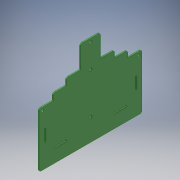
# Autodesk Inventor part: PCB
Saved by Autodesk Inventor 2017 (Build 210142000, 142)
## iProperties
Created: 2016-11-14
Part Number: PCB
Material: Generic
Document SubType Name: Modeling
Designer: Shichi
Density: 1 g/cm^3
Appearance: Smooth - Dark Forest Green
Author: Shichi
Autodesk Inventor part; units mm, degrees
ref_plane "YZ Plane" through (0, 0, 0) normal (1, 0, 0) x (0, 1, 0)
ref_plane "XZ Plane" through (0, 0, 0) normal (0, 1, 0) x (-1, 0, 0)
ref_plane "XY Plane" through (0, 0, 0) normal (0, 0, 1) x (1, 0, 0)
sketch "Sketch1" plane through (0, 0, 0) normal (1, 0, 0) x (0, 1, 0)
  line L0 (47, 25) -> (-47, 25)
  line L1 (-47, 25) -> (-47, -25)
  line L2 (-47, -25) -> (47, -25)
  line L3 (47, -25) -> (47, 25)
  circle A0 centre (44, 22) radius 1.25
  line L4 (0, 25) -> (0, -25) construction
  circle A1 centre (-44, 22) radius 1.25
  line L5 (-34, 25) -> (-34, 31)
  line L6 (-34, 31) -> (34, 31)
  line L7 (34, 31) -> (34, 25)
  line L8 (-33, -12) -> (-22, -12)
  line L9 (-22, -12) -> (-22, -13)
  line L10 (-22, -13) -> (-33, -13)
  line L11 (-33, -13) -> (-33, -12)
  line L12 (33, -12) -> (22, -12)
  line L13 (22, -12) -> (22, -13)
  line L14 (22, -13) -> (33, -13)
  line L15 (33, -13) -> (33, -12)
  line L16 (-41, 7) -> (-42, 7)
  line L17 (-42, 7) -> (-42, -4)
  line L18 (-42, -4) -> (-41, -4)
  line L19 (-41, -4) -> (-41, 7)
  line L20 (41, 7) -> (42, 7)
  line L21 (42, 7) -> (42, -4)
  line L22 (42, -4) -> (41, -4)
  line L23 (41, -4) -> (41, 7)
  circle A2 centre (0, -5) radius 1.25
  circle A3 centre (0, 54.3) radius 1.25
  line L24 (22, 31) -> (22, 37)
  line L25 (22, 37) -> (9, 37)
  line L26 (9, 37) -> (9, 57.5)
  line L27 (-9, 57.5) -> (-9, 37)
  line L28 (-9, 37) -> (-22, 37)
  line L29 (-22, 37) -> (-22, 31)
  line L30 (9, 57.5) -> (-9, 57.5)
  circle A4 centre (0, 32.7) radius 1.25
  point P0 (0, 0)
  point P1 (47, 0)
  dimension "d0" = 50
  dimension "d1" = 94
  dimension "d2" = 2.5
  dimension "d3" = 3
  dimension "d4" = 3
  dimension "d11" = 13
  dimension "d12" = 6
  dimension "d13" = 13
  dimension "d18" = 1
  dimension "d19" = 11
  dimension "d20" = 14
  dimension "d21" = 12
  dimension "d24" = 21
  dimension "d25" = 1
  dimension "d26" = 5
  dimension "d27" = 11
  dimension "d28" = 30
  dimension "d29" = 2.5
  dimension "d30" = 2.5
  dimension "d33" = 6
  dimension "d34" = 25
  dimension "d35" = 25
  dimension "d37" = 12
  dimension "d38" = 12
  dimension "d39" = 9
  dimension "d41" = 26.5
  dimension "d42" = 3.2
  dimension "d43" = 2.5
  dimension "d44" = 37.7
  constraints: 62 end point, 9 perpendicular, 9 symmetric about line, 8 point on line, 7 parallel, 5 centre point, 5 horizontal, 3 midpoint, 3 vertical alignment, 2 horizontal alignment, 1 other
  measures "d0" distance of L2.end L0.start
  measures "d1" distance of L1.end L2.end
  measures "d2" diameter of A0
  measures "d3" distance from line of A0.centre L3
  measures "d4" distance from line of L0 A0.centre
  measures "d11" distance from line of L0.end L5
  measures "d12" distance of L5.start L5.end
  measures "d13" distance from line of L7 L0.start
  measures "d18" distance between parallel lines of L10 L8
  measures "d19" distance between parallel lines of L9 L11
  measures "d20" distance from line of L1 L8.start
  measures "d21" distance between parallel lines of L2 L10
  measures "d24" distance between parallel lines of L18 L2
  measures "d25" distance between parallel lines of L19 L17
  measures "d26" distance between parallel lines of L1 L17
  measures "d27" distance of L18.end L16.start
  measures "d28" distance from line of L0 A2.centre
  measures "d29" diameter of A2
  measures "d30" diameter of A3
  measures "d33" distance of L24.start L24.end
  measures "d34" distance between parallel lines of L7 L26
  measures "d35" distance between parallel lines of L5 L27
  measures "d37" distance between parallel lines of L7 L24
  measures "d38" distance between parallel lines of L5 L29
  measures "d39" distance from line of L27 A3.centre
  measures "d41" distance between parallel lines of L6 L30
  measures "d42" distance from line of L30 A3.centre
  measures "d43" diameter of A4
  measures "d44" distance of A2.centre A4.centre
extrude "Extrusion1" add sketch "Sketch1" along normal blind 1 contours L3 L2 L1 L0 | L0 L5 L6 L7 | L6 L29 L28 L27 L30 L26 L25 L24 | L8 L9 L10 L11 | L15 L14 L13 L12 | L19 L18 L17 L16 | L20 L21 L22 L23 | A2 | A3 | A4
fillet "Fillet1" radius 2 10 edges at (0.5, -47, 25) (0.5, -34, 31) (0.5, 34, 31) (0.5, 47, 25) (0.5, -47, -25) (0.5, 47, -25) (0.5, 9, 57.5) (0.5, -9, 57.5) (0.5, 22, 37) (0.5, -22, 37)
extrude "Extrusion2" cut sketch "Sketch1" along normal up to next contours L8 L9 L10 L11 | L15 L14 L13 L12 | L19 L18 L17 L16 | L20 L21 L22 L23 | A2 | A3 | A4
body "Solid1"
